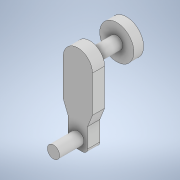
# Autodesk Inventor part: 2번부품
Saved by Autodesk Inventor 2022 (Build 260153000, 153)
## iProperties
Created: 2021-09-05
Part Number: 2번부품
Material: 일반
Document SubType Name: Modeling
Designer: 서울공업고등학교
Density: 1 g/cm^3
Appearance: 기본값
Author: 서울공업고등학교
Autodesk Inventor part; units mm, degrees
ref_plane "YZ Plane" through (0, 0, 0) normal (1, 0, 0) x (0, 1, 0)
ref_plane "XZ Plane" through (0, 0, 0) normal (0, 1, 0) x (-1, 0, 0)
ref_plane "XY Plane" through (0, 0, 0) normal (0, 0, 1) x (1, 0, 0)
sketch "스케치1" plane through (0, 0, 0) normal (0, 0, 1) x (1, 0, 0)
  circle A0 centre (0, 0) radius 2.5
  line L0 (0, 0) -> (0, 40)
  line L1 (4, 6) -> (4, -4)
  line L2 (4, -4) -> (-4, -4)
  line L3 (-4, -4) -> (-4, 6)
  line L4 (-6, 32) -> (6, 32)
  line L5 (6, 32) -> (6, 11)
  line L6 (-6, 11) -> (-6, 32)
  line L7 (-6, 11) -> (-4, 6)
  line L8 (6, 11) -> (4, 6)
  dimension "d0" = 5
  dimension "d1" = 40
  dimension "d2" = 8
  dimension "d3" = 4
  dimension "d4" = 4
  dimension "d5" = 36
  dimension "d8" = 12
  dimension "d9" = 6
  dimension "d10" = 10
  dimension "d11" = 5
  dimension "d12" = 5
  dimension "d13" = 10
  constraints: 18 end point, 2 parallel, 1 centre point, 1 coincident, 1 horizontal, 1 horizontal alignment, 1 perpendicular, 1 vertical
  measures "d0" diameter of A0
  measures "d1" distance of L0.start L0.end
  measures "d2" distance between parallel lines of L1 L3
  measures "d3" distance from line of point (0, 0) L2
  measures "d4" distance from line of point (0, 0) L3
  measures "d5" distance between parallel lines of L2 L4
  measures "d8" distance between parallel lines of L5 L6
  measures "d9" distance from line of point (0, 0) L6
  measures "d10" distance of L2.end L3.end
  measures "d11" vertical distance of L6.start L3.end
  measures "d12" vertical distance of L5.end L1.start
  measures "d13" distance from line of L2 L1.start
extrude "돌출1" add sketch "스케치1" along normal blind 5
extrude "돌출2" add sketch "스케치1" along normal blind 15 contours A0
sketch "스케치2" plane through (0, 0, 0) normal (0, 0, -1) x (-1, 0, 0)
  circle A0 centre (0, 26) radius 2.5
  line L0 (-6, 11) -> (-6, 32) projected
  line L1 (4, -4) -> (-4, -4) projected
  point P0 (0, 0)
  dimension "d18" = 5
  dimension "d19" = 6
  dimension "d20" = 30
  constraints: 1 centre point
  measures "d18" diameter of A0
  measures "d19" distance from line of A0.centre L0
  measures "d20" distance from line of L1 A0.centre
extrude "돌출3" add sketch "스케치2" along normal blind 11
sketch "스케치3" plane through (0, 26, -11) normal (0, 0, -1) x (-1, 0, 0)
  circle A0 centre (0, 0) radius 7
  point P0 (0, -26)
  dimension "d23" = 14
  constraints: 1 centre point
  measures "d23" diameter of A0
extrude "돌출4" add sketch "스케치3" along normal blind 4
fillet "모깎기1" radius 2 2 edges at (-4, -4, 2.5) (4, -4, 2.5)
fillet "모깎기2" radius 6 2 edges at (6, 32, 2.5) (-6, 32, 2.5)
